Autodesk Inventor part; units mm, degrees
(part 5 of 6)
  line L3382 (247.1746, 190.2602) -> (246.7243, 190.3176)
  line L3383 (246.7243, 190.3176) -> (246.2809, 190.3966)
  line L3384 (246.2809, 190.3966) -> (245.8455, 190.4972)
  line L3385 (245.8455, 190.4972) -> (245.4186, 190.6185)
  line L3386 (245.4186, 190.6185) -> (245.0004, 190.7599)
  line L3387 (245.0004, 190.7599) -> (244.5914, 190.9212)
  line L3388 (244.5914, 190.9212) -> (244.1928, 191.1013)
  line L3389 (244.1928, 191.1013) -> (243.8049, 191.3001)
  line L3390 (243.8049, 191.3001) -> (243.428, 191.5168)
  line L3391 (243.428, 191.5168) -> (243.0629, 191.7509)
  line L3392 (243.0629, 191.7509) -> (242.7101, 192.0019)
  line L3393 (242.7101, 192.0019) -> (242.37, 192.2691)
  line L3394 (242.37, 192.2691) -> (242.0435, 192.5519)
  line L3395 (242.0435, 192.5519) -> (241.7306, 192.8499)
  line L3396 (241.7306, 192.8499) -> (241.433, 193.1624)
  line L3397 (241.433, 193.1624) -> (241.1498, 193.489)
  line L3398 (241.1498, 193.489) -> (240.8828, 193.829)
  line L3399 (240.8828, 193.829) -> (240.632, 194.1818)
  line L3400 (240.632, 194.1818) -> (240.3977, 194.547)
  line L3401 (240.3977, 194.547) -> (240.181, 194.9238)
  line L3402 (240.181, 194.9238) -> (239.9823, 195.3119)
  line L3403 (239.9823, 195.3119) -> (239.8021, 195.7107)
  line L3404 (239.8021, 195.7107) -> (239.6408, 196.1193)
  line L3405 (239.6408, 196.1193) -> (239.4992, 196.5375)
  line L3406 (239.4992, 196.5375) -> (239.378, 196.9645)
  line L3407 (239.378, 196.9645) -> (239.2777, 197.4)
  line L3408 (239.2777, 197.4) -> (239.1985, 197.8432)
  line L3409 (239.1985, 197.8432) -> (239.1413, 198.2937)
  line L3410 (239.1413, 198.2937) -> (239.1065, 198.7507)
  line L3411 (239.1065, 198.7507) -> (239.0948, 199.2139)
  line L3412 (239.0948, 171.1778) -> (239.1065, 171.641)
  line L3413 (239.1065, 171.641) -> (239.1413, 172.098)
  line L3414 (239.1413, 172.098) -> (239.1985, 172.5485)
  line L3415 (239.1985, 172.5485) -> (239.2777, 172.9917)
  line L3416 (239.2777, 172.9917) -> (239.378, 173.4271)
  line L3417 (239.378, 173.4271) -> (239.4992, 173.8542)
  line L3418 (239.4992, 173.8542) -> (239.6408, 174.2724)
  line L3419 (239.6408, 174.2724) -> (239.8021, 174.681)
  line L3420 (239.8021, 174.681) -> (239.9823, 175.0798)
  line L3421 (239.9823, 175.0798) -> (240.181, 175.4678)
  line L3422 (240.181, 175.4678) -> (240.3977, 175.8447)
  line L3423 (240.3977, 175.8447) -> (240.632, 176.2097)
  line L3424 (240.632, 176.2097) -> (240.8828, 176.5627)
  line L3425 (240.8828, 176.5627) -> (241.1498, 176.9027)
  line L3426 (241.1498, 176.9027) -> (241.433, 177.2291)
  line L3427 (241.433, 177.2291) -> (241.7306, 177.5418)
  line L3428 (241.7306, 177.5418) -> (242.0435, 177.8398)
  line L3429 (242.0435, 177.8398) -> (242.37, 178.1226)
  line L3430 (242.37, 178.1226) -> (242.7101, 178.3898)
  line L3431 (242.7101, 178.3898) -> (243.0629, 178.6408)
  line L3432 (243.0629, 178.6408) -> (243.428, 178.8749)
  line L3433 (243.428, 178.8749) -> (243.8049, 179.0916)
  line L3434 (243.8049, 179.0916) -> (244.1928, 179.2903)
  line L3435 (244.1928, 179.2903) -> (244.5914, 179.4705)
  line L3436 (244.5914, 179.4705) -> (245.0004, 179.6318)
  line L3437 (245.0004, 179.6318) -> (245.4186, 179.7732)
  line L3438 (245.4186, 179.7732) -> (245.8455, 179.8944)
  line L3439 (245.8455, 179.8944) -> (246.2809, 179.995)
  line L3440 (246.2809, 179.995) -> (246.7243, 180.0741)
  line L3441 (246.7243, 180.0741) -> (247.1746, 180.1313)
  line L3442 (247.1746, 180.1313) -> (247.6317, 180.1661)
  line L3443 (247.6317, 180.1661) -> (248.0948, 180.1778)
  line L3444 (248.0948, 180.1778) -> (248.5578, 180.1661)
  line L3445 (248.5578, 180.1661) -> (249.0149, 180.1313)
  line L3446 (249.0149, 180.1313) -> (249.4656, 180.0741)
  line L3447 (249.4656, 180.0741) -> (249.9086, 179.995)
  line L3448 (249.9086, 179.995) -> (250.3441, 179.8944)
  line L3449 (250.3441, 179.8944) -> (250.7713, 179.7732)
  line L3450 (250.7713, 179.7732) -> (251.1891, 179.6318)
  line L3451 (251.1891, 179.6318) -> (251.5981, 179.4705)
  line L3452 (251.5981, 179.4705) -> (251.9967, 179.2903)
  line L3453 (251.9967, 179.2903) -> (252.3846, 179.0916)
  line L3454 (252.3846, 179.0916) -> (252.7615, 178.8749)
  line L3455 (252.7615, 178.8749) -> (253.1267, 178.6408)
  line L3456 (253.1267, 178.6408) -> (253.4798, 178.3898)
  line L3457 (253.4798, 178.3898) -> (253.8195, 178.1226)
  line L3458 (253.8195, 178.1226) -> (254.1461, 177.8398)
  line L3459 (254.1461, 177.8398) -> (254.4589, 177.5418)
  line L3460 (254.4589, 177.5418) -> (254.7569, 177.2291)
  line L3461 (254.7569, 177.2291) -> (255.0397, 176.9027)
  line L3462 (255.0397, 176.9027) -> (255.3067, 176.5627)
  line L3463 (255.3067, 176.5627) -> (255.5579, 176.2097)
  line L3464 (255.5579, 176.2097) -> (255.7918, 175.8447)
  line L3465 (255.7918, 175.8447) -> (256.0085, 175.4678)
  line L3466 (256.0085, 175.4678) -> (256.2073, 175.0798)
  line L3467 (256.2073, 175.0798) -> (256.3875, 174.681)
  line L3468 (256.3875, 174.681) -> (256.5487, 174.2724)
  line L3469 (256.5487, 174.2724) -> (256.6903, 173.8542)
  line L3470 (256.6903, 173.8542) -> (256.8115, 173.4271)
  line L3471 (256.8115, 173.4271) -> (256.9118, 172.9917)
  line L3472 (256.9118, 172.9917) -> (256.991, 172.5485)
  line L3473 (256.991, 172.5485) -> (257.0482, 172.098)
  line L3474 (257.0482, 172.098) -> (257.083, 171.641)
  line L3475 (257.083, 171.641) -> (257.0947, 171.1778)
  line L3476 (257.0947, 171.1778) -> (257.083, 170.7146)
  line L3477 (257.083, 170.7146) -> (257.0482, 170.2577)
  line L3478 (257.0482, 170.2577) -> (256.991, 169.8072)
  line L3479 (256.991, 169.8072) -> (256.9118, 169.364)
  line L3480 (256.9118, 169.364) -> (256.8115, 168.9285)
  line L3481 (256.8115, 168.9285) -> (256.6903, 168.5015)
  line L3482 (256.6903, 168.5015) -> (256.5487, 168.0833)
  line L3483 (256.5487, 168.0833) -> (256.3875, 167.6747)
  line L3484 (256.3875, 167.6747) -> (256.2073, 167.2759)
  line L3485 (256.2073, 167.2759) -> (256.0085, 166.8878)
  line L3486 (256.0085, 166.8878) -> (255.7918, 166.5109)
  line L3487 (255.7918, 166.5109) -> (255.5579, 166.1459)
  line L3488 (255.5579, 166.1459) -> (255.3067, 165.793)
  line L3489 (255.3067, 165.793) -> (255.0397, 165.4529)
  line L3490 (255.0397, 165.4529) -> (254.7569, 165.1265)
  line L3491 (254.7569, 165.1265) -> (254.4589, 164.8139)
  line L3492 (254.4589, 164.8139) -> (254.1461, 164.5159)
  line L3493 (254.1461, 164.5159) -> (253.8195, 164.233)
  line L3494 (253.8195, 164.233) -> (253.4798, 163.9659)
  line L3495 (253.4798, 163.9659) -> (253.1267, 163.7149)
  line L3496 (253.1267, 163.7149) -> (252.7615, 163.4808)
  line L3497 (252.7615, 163.4808) -> (252.3846, 163.2641)
  line L3498 (252.3846, 163.2641) -> (251.9967, 163.0653)
  line L3499 (251.9967, 163.0653) -> (251.5981, 162.8851)
  line L3500 (251.5981, 162.8851) -> (251.1891, 162.7239)
  line L3501 (251.1891, 162.7239) -> (250.7713, 162.5825)
  line L3502 (250.7713, 162.5825) -> (250.3441, 162.4612)
  line L3503 (250.3441, 162.4612) -> (249.9086, 162.3606)
  line L3504 (249.9086, 162.3606) -> (249.4656, 162.2816)
  line L3505 (249.4656, 162.2816) -> (249.0149, 162.2244)
  line L3506 (249.0149, 162.2244) -> (248.5578, 162.1896)
  line L3507 (248.5578, 162.1896) -> (248.0948, 162.1779)
  line L3508 (248.0948, 162.1779) -> (247.6317, 162.1896)
  line L3509 (247.6317, 162.1896) -> (247.1746, 162.2244)
  line L3510 (247.1746, 162.2244) -> (246.7243, 162.2816)
  line L3511 (246.7243, 162.2816) -> (246.2809, 162.3606)
  line L3512 (246.2809, 162.3606) -> (245.8455, 162.4612)
  line L3513 (245.8455, 162.4612) -> (245.4186, 162.5825)
  line L3514 (245.4186, 162.5825) -> (245.0004, 162.7239)
  line L3515 (245.0004, 162.7239) -> (244.5914, 162.8851)
  line L3516 (244.5914, 162.8851) -> (244.1928, 163.0653)
  line L3517 (244.1928, 163.0653) -> (243.8049, 163.2641)
  line L3518 (243.8049, 163.2641) -> (243.428, 163.4808)
  line L3519 (243.428, 163.4808) -> (243.0629, 163.7149)
  line L3520 (243.0629, 163.7149) -> (242.7101, 163.9659)
  line L3521 (242.7101, 163.9659) -> (242.37, 164.233)
  line L3522 (242.37, 164.233) -> (242.0435, 164.5159)
  line L3523 (242.0435, 164.5159) -> (241.7306, 164.8139)
  line L3524 (241.7306, 164.8139) -> (241.433, 165.1265)
  line L3525 (241.433, 165.1265) -> (241.1498, 165.4529)
  line L3526 (241.1498, 165.4529) -> (240.8828, 165.793)
  line L3527 (240.8828, 165.793) -> (240.632, 166.1459)
  line L3528 (240.632, 166.1459) -> (240.3977, 166.5109)
  line L3529 (240.3977, 166.5109) -> (240.181, 166.8878)
  line L3530 (240.181, 166.8878) -> (239.9823, 167.2759)
  line L3531 (239.9823, 167.2759) -> (239.8021, 167.6747)
  line L3532 (239.8021, 167.6747) -> (239.6408, 168.0833)
  line L3533 (239.6408, 168.0833) -> (239.4992, 168.5015)
  line L3534 (239.4992, 168.5015) -> (239.378, 168.9285)
  line L3535 (239.378, 168.9285) -> (239.2777, 169.364)
  line L3536 (239.2777, 169.364) -> (239.1985, 169.8072)
  line L3537 (239.1985, 169.8072) -> (239.1413, 170.2577)
  line L3538 (239.1413, 170.2577) -> (239.1065, 170.7146)
  line L3539 (239.1065, 170.7146) -> (239.0948, 171.1778)
  line L3540 (242.0924, 148.6958) -> (242.1003, 149.0045)
  line L3541 (242.1003, 149.0045) -> (242.1234, 149.3092)
  line L3542 (242.1234, 149.3092) -> (242.1616, 149.6096)
  line L3543 (242.1616, 149.6096) -> (242.2143, 149.9051)
  line L3544 (242.2143, 149.9051) -> (242.3621, 150.48)
  line L3545 (242.3621, 150.48) -> (242.564, 151.0313)
  line L3546 (242.564, 151.0313) -> (242.8165, 151.5558)
  line L3547 (242.8165, 151.5558) -> (243.1169, 152.0505)
  line L3548 (243.1169, 152.0505) -> (243.4625, 152.5123)
  line L3549 (243.4625, 152.5123) -> (243.8497, 152.9385)
  line L3550 (243.8497, 152.9385) -> (244.2759, 153.3257)
  line L3551 (244.2759, 153.3257) -> (244.7379, 153.6711)
  line L3552 (244.7379, 153.6711) -> (245.2326, 153.9717)
  line L3553 (245.2326, 153.9717) -> (245.7569, 154.2244)
  line L3554 (245.7569, 154.2244) -> (246.3081, 154.4261)
  line L3555 (246.3081, 154.4261) -> (246.8831, 154.5739)
  line L3556 (246.8831, 154.5739) -> (247.1787, 154.6267)
  line L3557 (247.1787, 154.6267) -> (247.4788, 154.6648)
  line L3558 (247.4788, 154.6648) -> (247.7837, 154.6881)
  line L3559 (247.7837, 154.6881) -> (248.0924, 154.6958)
  line L3560 (248.0924, 154.6958) -> (248.401, 154.6881)
  line L3561 (248.401, 154.6881) -> (248.7059, 154.6648)
  line L3562 (248.7059, 154.6648) -> (249.006, 154.6267)
  line L3563 (249.006, 154.6267) -> (249.3016, 154.5739)
  line L3564 (249.3016, 154.5739) -> (249.8766, 154.4261)
  line L3565 (249.8766, 154.4261) -> (250.4278, 154.2244)
  line L3566 (250.4278, 154.2244) -> (250.9525, 153.9717)
  line L3567 (250.9525, 153.9717) -> (251.4472, 153.6711)
  line L3568 (251.4472, 153.6711) -> (251.9088, 153.3257)
  line L3569 (251.9088, 153.3257) -> (252.335, 152.9385)
  line L3570 (252.335, 152.9385) -> (252.7222, 152.5123)
  line L3571 (252.7222, 152.5123) -> (253.0678, 152.0505)
  line L3572 (253.0678, 152.0505) -> (253.3682, 151.5558)
  line L3573 (253.3682, 151.5558) -> (253.621, 151.0313)
  line L3574 (253.621, 151.0313) -> (253.8226, 150.48)
  line L3575 (253.8226, 150.48) -> (253.9704, 149.9051)
  line L3576 (253.9704, 149.9051) -> (254.0234, 149.6096)
  line L3577 (254.0234, 149.6096) -> (254.0613, 149.3092)
  line L3578 (254.0613, 149.3092) -> (254.0847, 149.0045)
  line L3579 (254.0847, 149.0045) -> (254.0923, 148.6958)
  line L3580 (254.0923, 148.6958) -> (254.0847, 148.3872)
  line L3581 (254.0847, 148.3872) -> (254.0613, 148.0823)
  line L3582 (254.0613, 148.0823) -> (254.0234, 147.7822)
  line L3583 (254.0234, 147.7822) -> (253.9704, 147.4866)
  line L3584 (253.9704, 147.4866) -> (253.8226, 146.9116)
  line L3585 (253.8226, 146.9116) -> (253.621, 146.3604)
  line L3586 (253.621, 146.3604) -> (253.3682, 145.8357)
  line L3587 (253.3682, 145.8357) -> (253.0678, 145.341)
  line L3588 (253.0678, 145.341) -> (252.7222, 144.8794)
  line L3589 (252.7222, 144.8794) -> (252.335, 144.4532)
  line L3590 (252.335, 144.4532) -> (251.9088, 144.066)
  line L3591 (251.9088, 144.066) -> (251.4472, 143.7204)
  line L3592 (251.4472, 143.7204) -> (250.9525, 143.42)
  line L3593 (250.9525, 143.42) -> (250.4278, 143.1675)
  line L3594 (250.4278, 143.1675) -> (249.8766, 142.9656)
  line L3595 (249.8766, 142.9656) -> (249.3016, 142.8178)
  line L3596 (249.3016, 142.8178) -> (249.006, 142.7651)
  line L3597 (249.006, 142.7651) -> (248.7059, 142.7269)
  line L3598 (248.7059, 142.7269) -> (248.401, 142.7038)
  line L3599 (248.401, 142.7038) -> (248.0924, 142.6959)
  line L3600 (248.0924, 142.6959) -> (247.7837, 142.7038)
  line L3601 (247.7837, 142.7038) -> (247.4788, 142.7269)
  line L3602 (247.4788, 142.7269) -> (247.1787, 142.7651)
  line L3603 (247.1787, 142.7651) -> (246.8831, 142.8178)
  line L3604 (246.8831, 142.8178) -> (246.3081, 142.9656)
  line L3605 (246.3081, 142.9656) -> (245.7569, 143.1675)
  line L3606 (245.7569, 143.1675) -> (245.2326, 143.42)
  line L3607 (245.2326, 143.42) -> (244.7379, 143.7204)
  line L3608 (244.7379, 143.7204) -> (244.2759, 144.066)
  line L3609 (244.2759, 144.066) -> (243.8497, 144.4532)
  line L3610 (243.8497, 144.4532) -> (243.4625, 144.8794)
  line L3611 (243.4625, 144.8794) -> (243.1169, 145.341)
  line L3612 (243.1169, 145.341) -> (242.8165, 145.8357)
  line L3613 (242.8165, 145.8357) -> (242.564, 146.3604)
  line L3614 (242.564, 146.3604) -> (242.3621, 146.9116)
  line L3615 (242.3621, 146.9116) -> (242.2143, 147.4866)
  line L3616 (242.2143, 147.4866) -> (242.1616, 147.7822)
  line L3617 (242.1616, 147.7822) -> (242.1234, 148.0823)
  line L3618 (242.1234, 148.0823) -> (242.1003, 148.3872)
  line L3619 (242.1003, 148.3872) -> (242.0924, 148.6958)
  line L3620 (239.0948, 126.1997) -> (239.1065, 126.6631)
  line L3621 (239.1065, 126.6631) -> (239.1413, 127.1199)
  line L3622 (239.1413, 127.1199) -> (239.1985, 127.5705)
  line L3623 (239.1985, 127.5705) -> (239.2777, 128.0135)
  line L3624 (239.2777, 128.0135) -> (239.378, 128.449)
  line L3625 (239.378, 128.449) -> (239.4992, 128.8762)
  line L3626 (239.4992, 128.8762) -> (239.6408, 129.2944)
  line L3627 (239.6408, 129.2944) -> (239.8021, 129.703)
  line L3628 (239.8021, 129.703) -> (239.9823, 130.1016)
  line L3629 (239.9823, 130.1016) -> (240.181, 130.4899)
  line L3630 (240.181, 130.4899) -> (240.3977, 130.8668)
  line L3631 (240.3977, 130.8668) -> (240.632, 131.232)
  line L3632 (240.632, 131.232) -> (240.8828, 131.5847)
  line L3633 (240.8828, 131.5847) -> (241.1498, 131.9248)
  line L3634 (241.1498, 131.9248) -> (241.433, 132.2514)
  line L3635 (241.433, 132.2514) -> (241.7306, 132.5638)
  line L3636 (241.7306, 132.5638) -> (242.0435, 132.8618)
  line L3637 (242.0435, 132.8618) -> (242.37, 133.1447)
  line L3638 (242.37, 133.1447) -> (242.7101, 133.412)
  line L3639 (242.7101, 133.412) -> (243.0629, 133.6628)
  line L3640 (243.0629, 133.6628) -> (243.428, 133.8967)
  line L3641 (243.428, 133.8967) -> (243.8049, 134.1134)
  line L3642 (243.8049, 134.1134) -> (244.1928, 134.3122)
  line L3643 (244.1928, 134.3122) -> (244.5914, 134.4924)
  line L3644 (244.5914, 134.4924) -> (245.0004, 134.6536)
  line L3645 (245.0004, 134.6536) -> (245.4186, 134.7952)
  line L3646 (245.4186, 134.7952) -> (245.8455, 134.9165)
  line L3647 (245.8455, 134.9165) -> (246.2809, 135.0171)
  line L3648 (246.2809, 135.0171) -> (246.7243, 135.096)
  line L3649 (246.7243, 135.096) -> (247.1746, 135.1535)
  line L3650 (247.1746, 135.1535) -> (247.6317, 135.188)
  line L3651 (247.6317, 135.188) -> (248.0948, 135.1997)
  line L3652 (248.0948, 135.1997) -> (248.5578, 135.188)
  line L3653 (248.5578, 135.188) -> (249.0149, 135.1535)
  line L3654 (249.0149, 135.1535) -> (249.4656, 135.096)
  line L3655 (249.4656, 135.096) -> (249.9086, 135.0171)
  line L3656 (249.9086, 135.0171) -> (250.3441, 134.9165)
  line L3657 (250.3441, 134.9165) -> (250.7713, 134.7952)
  line L3658 (250.7713, 134.7952) -> (251.1891, 134.6536)
  line L3659 (251.1891, 134.6536) -> (251.5981, 134.4924)
  line L3660 (251.5981, 134.4924) -> (251.9967, 134.3122)
  line L3661 (251.9967, 134.3122) -> (252.3846, 134.1134)
  line L3662 (252.3846, 134.1134) -> (252.7615, 133.8967)
  line L3663 (252.7615, 133.8967) -> (253.1267, 133.6628)
  line L3664 (253.1267, 133.6628) -> (253.4798, 133.412)
  line L3665 (253.4798, 133.412) -> (253.8195, 133.1447)
  line L3666 (253.8195, 133.1447) -> (254.1461, 132.8618)
  line L3667 (254.1461, 132.8618) -> (254.4589, 132.5638)
  line L3668 (254.4589, 132.5638) -> (254.7569, 132.2514)
  line L3669 (254.7569, 132.2514) -> (255.0397, 131.9248)
  line L3670 (255.0397, 131.9248) -> (255.3067, 131.5847)
  line L3671 (255.3067, 131.5847) -> (255.5579, 131.232)
  line L3672 (255.5579, 131.232) -> (255.7918, 130.8668)
  line L3673 (255.7918, 130.8668) -> (256.0085, 130.4899)
  line L3674 (256.0085, 130.4899) -> (256.2073, 130.1016)
  line L3675 (256.2073, 130.1016) -> (256.3875, 129.703)
  line L3676 (256.3875, 129.703) -> (256.5487, 129.2944)
  line L3677 (256.5487, 129.2944) -> (256.6903, 128.8762)
  line L3678 (256.6903, 128.8762) -> (256.8115, 128.449)
  line L3679 (256.8115, 128.449) -> (256.9118, 128.0135)
  line L3680 (256.9118, 128.0135) -> (256.991, 127.5705)
  line L3681 (256.991, 127.5705) -> (257.0482, 127.1199)
  line L3682 (257.0482, 127.1199) -> (257.083, 126.6631)
  line L3683 (257.083, 126.6631) -> (257.0947, 126.1997)
  line L3684 (257.0947, 126.1997) -> (257.083, 125.7367)
  line L3685 (257.083, 125.7367) -> (257.0482, 125.2795)
  line L3686 (257.0482, 125.2795) -> (256.991, 124.8292)
  line L3687 (256.991, 124.8292) -> (256.9118, 124.3859)
  line L3688 (256.9118, 124.3859) -> (256.8115, 123.9507)
  line L3689 (256.8115, 123.9507) -> (256.6903, 123.5236)
  line L3690 (256.6903, 123.5236) -> (256.5487, 123.1053)
  line L3691 (256.5487, 123.1053) -> (256.3875, 122.6967)
  line L3692 (256.3875, 122.6967) -> (256.2073, 122.2981)
  line L3693 (256.2073, 122.2981) -> (256.0085, 121.9099)
  line L3694 (256.0085, 121.9099) -> (255.7918, 121.533)
  line L3695 (255.7918, 121.533) -> (255.5579, 121.1678)
  line L3696 (255.5579, 121.1678) -> (255.3067, 120.815)
  line L3697 (255.3067, 120.815) -> (255.0397, 120.475)
  line L3698 (255.0397, 120.475) -> (254.7569, 120.1484)
  line L3699 (254.7569, 120.1484) -> (254.4589, 119.8359)
  line L3700 (254.4589, 119.8359) -> (254.1461, 119.5379)
  line L3701 (254.1461, 119.5379) -> (253.8195, 119.2551)
  line L3702 (253.8195, 119.2551) -> (253.4798, 118.9877)
  line L3703 (253.4798, 118.9877) -> (253.1267, 118.7369)
  line L3704 (253.1267, 118.7369) -> (252.7615, 118.5027)
  line L3705 (252.7615, 118.5027) -> (252.3846, 118.286)
  line L3706 (252.3846, 118.286) -> (251.9967, 118.0872)
  line L3707 (251.9967, 118.0872) -> (251.5981, 117.907)
  line L3708 (251.5981, 117.907) -> (251.1891, 117.7458)
  line L3709 (251.1891, 117.7458) -> (250.7713, 117.6045)
  line L3710 (250.7713, 117.6045) -> (250.3441, 117.4833)
  line L3711 (250.3441, 117.4833) -> (249.9086, 117.3827)
  line L3712 (249.9086, 117.3827) -> (249.4656, 117.3034)
  line L3713 (249.4656, 117.3034) -> (249.0149, 117.2462)
  line L3714 (249.0149, 117.2462) -> (248.5578, 117.2115)
  line L3715 (248.5578, 117.2115) -> (248.0948, 117.1997)
  line L3716 (248.0948, 117.1997) -> (247.6317, 117.2115)
  line L3717 (247.6317, 117.2115) -> (247.1746, 117.2462)
  line L3718 (247.1746, 117.2462) -> (246.7243, 117.3034)
  line L3719 (246.7243, 117.3034) -> (246.2809, 117.3827)
  line L3720 (246.2809, 117.3827) -> (245.8455, 117.4833)
  line L3721 (245.8455, 117.4833) -> (245.4186, 117.6045)
  line L3722 (245.4186, 117.6045) -> (245.0004, 117.7458)
  line L3723 (245.0004, 117.7458) -> (244.5914, 117.907)
  line L3724 (244.5914, 117.907) -> (244.1928, 118.0872)
  line L3725 (244.1928, 118.0872) -> (243.8049, 118.286)
  line L3726 (243.8049, 118.286) -> (243.428, 118.5027)
  line L3727 (243.428, 118.5027) -> (243.0629, 118.7369)
  line L3728 (243.0629, 118.7369) -> (242.7101, 118.9877)
  line L3729 (242.7101, 118.9877) -> (242.37, 119.2551)
  line L3730 (242.37, 119.2551) -> (242.0435, 119.5379)
  line L3731 (242.0435, 119.5379) -> (241.7306, 119.8359)
  line L3732 (241.7306, 119.8359) -> (241.433, 120.1484)
  line L3733 (241.433, 120.1484) -> (241.1498, 120.475)
  line L3734 (241.1498, 120.475) -> (240.8828, 120.815)
  line L3735 (240.8828, 120.815) -> (240.632, 121.1678)
  line L3736 (240.632, 121.1678) -> (240.3977, 121.533)
  line L3737 (240.3977, 121.533) -> (240.181, 121.9099)
  line L3738 (240.181, 121.9099) -> (239.9823, 122.2981)
  line L3739 (239.9823, 122.2981) -> (239.8021, 122.6967)
  line L3740 (239.8021, 122.6967) -> (239.6408, 123.1053)
  line L3741 (239.6408, 123.1053) -> (239.4992, 123.5236)
  line L3742 (239.4992, 123.5236) -> (239.378, 123.9507)
  line L3743 (239.378, 123.9507) -> (239.2777, 124.3859)
  line L3744 (239.2777, 124.3859) -> (239.1985, 124.8292)
  line L3745 (239.1985, 124.8292) -> (239.1413, 125.2795)
  line L3746 (239.1413, 125.2795) -> (239.1065, 125.7367)
  line L3747 (239.1065, 125.7367) -> (239.0948, 126.1997)
  line L3748 (239.0755, 98.1797) -> (239.0872, 98.6431)
  line L3749 (239.0872, 98.6431) -> (239.122, 99.0999)
  line L3750 (239.122, 99.0999) -> (239.1792, 99.5505)
  line L3751 (239.1792, 99.5505) -> (239.2584, 99.9936)
  line L3752 (239.2584, 99.9936) -> (239.3587, 100.429)
  line L3753 (239.3587, 100.429) -> (239.48, 100.8562)
  line L3754 (239.48, 100.8562) -> (239.6215, 101.2744)
  line L3755 (239.6215, 101.2744) -> (239.7828, 101.683)
  line L3756 (239.7828, 101.683) -> (239.963, 102.0816)
  line L3757 (239.963, 102.0816) -> (240.1617, 102.4699)
  line L3758 (240.1617, 102.4699) -> (240.3784, 102.8468)
  line L3759 (240.3784, 102.8468) -> (240.6124, 103.212)
  line L3760 (240.6124, 103.212) -> (240.8635, 103.5647)
  line L3761 (240.8635, 103.5647) -> (241.1305, 103.9048)
  line L3762 (241.1305, 103.9048) -> (241.4133, 104.2314)
  line L3763 (241.4133, 104.2314) -> (241.7113, 104.5438)
  line L3764 (241.7113, 104.5438) -> (242.0242, 104.8418)
  line L3765 (242.0242, 104.8418) -> (242.3508, 105.1247)
  line L3766 (242.3508, 105.1247) -> (242.6904, 105.392)
  line L3767 (242.6904, 105.392) -> (243.0436, 105.6428)
  line L3768 (243.0436, 105.6428) -> (243.4084, 105.8767)
  line L3769 (243.4084, 105.8767) -> (243.7853, 106.0934)
  line L3770 (243.7853, 106.0934) -> (244.1736, 106.2922)
  line L3771 (244.1736, 106.2922) -> (244.5722, 106.4727)
  line L3772 (244.5722, 106.4727) -> (244.9807, 106.6336)
  line L3773 (244.9807, 106.6336) -> (245.399, 106.7752)
  line L3774 (245.399, 106.7752) -> (245.8262, 106.8965)
  line L3775 (245.8262, 106.8965) -> (246.2616, 106.9971)
  line L3776 (246.2616, 106.9971) -> (246.7047, 107.076)
  line L3777 (246.7047, 107.076) -> (247.1553, 107.1335)
  line L3778 (247.1553, 107.1335) -> (247.6121, 107.168)
  line L3779 (247.6121, 107.168) -> (248.0755, 107.1797)
  line L3780 (248.0755, 107.1797) -> (248.5385, 107.168)
  line L3781 (248.5385, 107.168) -> (248.9957, 107.1335)
  line L3782 (248.9957, 107.1335) -> (249.4459, 107.076)
  line L3783 (249.4459, 107.076) -> (249.8893, 106.9971)
  line L3784 (249.8893, 106.9971) -> (250.3248, 106.8965)
  line L3785 (250.3248, 106.8965) -> (250.7516, 106.7752)
  line L3786 (250.7516, 106.7752) -> (251.1699, 106.6336)
  line L3787 (251.1699, 106.6336) -> (251.5788, 106.4727)
  line L3788 (251.5788, 106.4727) -> (251.9774, 106.2922)
  line L3789 (251.9774, 106.2922) -> (252.3653, 106.0934)
  line L3790 (252.3653, 106.0934) -> (252.7422, 105.8767)
  line L3791 (252.7422, 105.8767) -> (253.1074, 105.6428)
  line L3792 (253.1074, 105.6428) -> (253.4602, 105.392)
  line L3793 (253.4602, 105.392) -> (253.8002, 105.1247)
  line L3794 (253.8002, 105.1247) -> (254.1268, 104.8418)
  line L3795 (254.1268, 104.8418) -> (254.4392, 104.5438)
  line L3796 (254.4392, 104.5438) -> (254.7373, 104.2314)
  line L3797 (254.7373, 104.2314) -> (255.0201, 103.9048)
  line L3798 (255.0201, 103.9048) -> (255.2874, 103.5647)
  line L3799 (255.2874, 103.5647) -> (255.5382, 103.212)
  line L3800 (255.5382, 103.212) -> (255.7725, 102.8468)
  line L3801 (255.7725, 102.8468) -> (255.9892, 102.4699)
  line L3802 (255.9892, 102.4699) -> (256.188, 102.0816)
  line L3803 (256.188, 102.0816) -> (256.3682, 101.683)
  line L3804 (256.3682, 101.683) -> (256.5294, 101.2744)
  line L3805 (256.5294, 101.2744) -> (256.6706, 100.8562)
  line L3806 (256.6706, 100.8562) -> (256.7919, 100.429)
  line L3807 (256.7919, 100.429) -> (256.8925, 99.9936)
  line L3808 (256.8925, 99.9936) -> (256.9717, 99.5505)
  line L3809 (256.9717, 99.5505) -> (257.0289, 99.0999)
  line L3810 (257.0289, 99.0999) -> (257.0637, 98.6431)
  line L3811 (257.0637, 98.6431) -> (257.0754, 98.1797)
  line L3812 (257.0754, 98.1797) -> (257.0637, 97.7167)
  line L3813 (257.0637, 97.7167) -> (257.0289, 97.2595)
  line L3814 (257.0289, 97.2595) -> (256.9717, 96.8093)
  line L3815 (256.9717, 96.8093) -> (256.8925, 96.3659)
  line L3816 (256.8925, 96.3659) -> (256.7919, 95.9308)
  line L3817 (256.7919, 95.9308) -> (256.6706, 95.5036)
  line L3818 (256.6706, 95.5036) -> (256.5294, 95.0853)
  line L3819 (256.5294, 95.0853) -> (256.3682, 94.6767)
  line L3820 (256.3682, 94.6767) -> (256.188, 94.2778)
  line L3821 (256.188, 94.2778) -> (255.9892, 93.8899)
  line L3822 (255.9892, 93.8899) -> (255.7725, 93.513)
  line L3823 (255.7725, 93.513) -> (255.5382, 93.1478)
  line L3824 (255.5382, 93.1478) -> (255.2874, 92.795)
  line L3825 (255.2874, 92.795) -> (255.0201, 92.455)
  line L3826 (255.0201, 92.455) -> (254.7373, 92.1284)
  line L3827 (254.7373, 92.1284) -> (254.4392, 91.8159)
  line L3828 (254.4392, 91.8159) -> (254.1268, 91.5179)
  line L3829 (254.1268, 91.5179) -> (253.8002, 91.2351)
  line L3830 (253.8002, 91.2351) -> (253.4602, 90.9677)
  line L3831 (253.4602, 90.9677) -> (253.1074, 90.7169)
  line L3832 (253.1074, 90.7169) -> (252.7422, 90.4827)
  line L3833 (252.7422, 90.4827) -> (252.3653, 90.266)
  line L3834 (252.3653, 90.266) -> (251.9774, 90.0672)
  line L3835 (251.9774, 90.0672) -> (251.5788, 89.887)
  line L3836 (251.5788, 89.887) -> (251.1699, 89.7258)
  line L3837 (251.1699, 89.7258) -> (250.7516, 89.5845)
  line L3838 (250.7516, 89.5845) -> (250.3248, 89.4633)
  line L3839 (250.3248, 89.4633) -> (249.8893, 89.3627)
  line L3840 (249.8893, 89.3627) -> (249.4459, 89.2834)
  line L3841 (249.4459, 89.2834) -> (248.9957, 89.2263)
  line L3842 (248.9957, 89.2263) -> (248.5385, 89.1915)
  line L3843 (248.5385, 89.1915) -> (248.0755, 89.1797)
  line L3844 (248.0755, 89.1797) -> (247.6121, 89.1915)
  line L3845 (247.6121, 89.1915) -> (247.1553, 89.2263)
  line L3846 (247.1553, 89.2263) -> (246.7047, 89.2834)
  line L3847 (246.7047, 89.2834) -> (246.2616, 89.3627)
  line L3848 (246.2616, 89.3627) -> (245.8262, 89.4633)
  line L3849 (245.8262, 89.4633) -> (245.399, 89.5845)
  line L3850 (245.399, 89.5845) -> (244.9807, 89.7258)
  line L3851 (244.9807, 89.7258) -> (244.5722, 89.887)
  line L3852 (244.5722, 89.887) -> (244.1736, 90.0672)
  line L3853 (244.1736, 90.0672) -> (243.7853, 90.266)
  line L3854 (243.7853, 90.266) -> (243.4084, 90.4827)
  line L3855 (243.4084, 90.4827) -> (243.0436, 90.7169)
  line L3856 (243.0436, 90.7169) -> (242.6904, 90.9677)
  line L3857 (242.6904, 90.9677) -> (242.3508, 91.2351)
  line L3858 (242.3508, 91.2351) -> (242.0242, 91.5179)
  line L3859 (242.0242, 91.5179) -> (241.7113, 91.8159)
  line L3860 (241.7113, 91.8159) -> (241.4133, 92.1284)
  line L3861 (241.4133, 92.1284) -> (241.1305, 92.455)
  line L3862 (241.1305, 92.455) -> (240.8635, 92.795)
  line L3863 (240.8635, 92.795) -> (240.6124, 93.1478)
  line L3864 (240.6124, 93.1478) -> (240.3784, 93.513)
  line L3865 (240.3784, 93.513) -> (240.1617, 93.8899)
  line L3866 (240.1617, 93.8899) -> (239.963, 94.2778)
  line L3867 (239.963, 94.2778) -> (239.7828, 94.6767)
  line L3868 (239.7828, 94.6767) -> (239.6215, 95.0853)
  line L3869 (239.6215, 95.0853) -> (239.48, 95.5036)
  line L3870 (239.48, 95.5036) -> (239.3587, 95.9308)
  line L3871 (239.3587, 95.9308) -> (239.2584, 96.3659)
  line L3872 (239.2584, 96.3659) -> (239.1792, 96.8093)
  line L3873 (239.1792, 96.8093) -> (239.122, 97.2595)
  line L3874 (239.122, 97.2595) -> (239.0872, 97.7167)
  line L3875 (239.0872, 97.7167) -> (239.0755, 98.1797)
  line L3876 (264.5279, 87.8958) -> (264.5437, 88.2127)
  line L3877 (264.5437, 88.2127) -> (264.5909, 88.5207)
  line L3878 (264.5909, 88.5207) -> (264.667, 88.8177)
  line L3879 (264.667, 88.8177) -> (264.7714, 89.1026)
  line L3880 (264.7714, 89.1026) -> (264.902, 89.3734)
  line L3881 (264.902, 89.3734) -> (265.0574, 89.629)
  line L3882 (265.0574, 89.629) -> (265.2358, 89.8677)
  line L3883 (265.2358, 89.8677) -> (265.4356, 90.0879)
  line L3884 (265.4356, 90.0879) -> (265.6558, 90.288)
  line L3885 (265.6558, 90.288) -> (265.8945, 90.4665)
  line L3886 (265.8945, 90.4665) -> (266.1502, 90.6215)
  line L3887 (266.1502, 90.6215) -> (266.4209, 90.7521)
  line L3888 (266.4209, 90.7521) -> (266.7059, 90.8565)
  line L3889 (266.7059, 90.8565) -> (267.0032, 90.933)
  line L3890 (267.0032, 90.933) -> (267.3108, 90.9798)
  line L3891 (267.3108, 90.9798) -> (267.6278, 90.996)
  line L3892 (267.6278, 90.996) -> (267.9447, 90.9798)
  line L3893 (267.9447, 90.9798) -> (268.2524, 90.933)
  line L3894 (268.2524, 90.933) -> (268.5497, 90.8565)
  line L3895 (268.5497, 90.8565) -> (268.8346, 90.7521)
  line L3896 (268.8346, 90.7521) -> (269.1054, 90.6215)
  line L3897 (269.1054, 90.6215) -> (269.361, 90.4665)
  line L3898 (269.361, 90.4665) -> (269.5997, 90.288)
  line L3899 (269.5997, 90.288) -> (269.8199, 90.0879)
  line L3900 (269.8199, 90.0879) -> (270.02, 89.8677)
  line L3901 (270.02, 89.8677) -> (270.1985, 89.629)
  line L3902 (270.1985, 89.629) -> (270.3535, 89.3734)
  line L3903 (270.3535, 89.3734) -> (270.4841, 89.1026)
  line L3904 (270.4841, 89.1026) -> (270.5885, 88.8177)
  line L3905 (270.5885, 88.8177) -> (270.6646, 88.5207)
  line L3906 (270.6646, 88.5207) -> (270.7118, 88.2127)
  line L3907 (270.7118, 88.2127) -> (270.7277, 87.8958)
  line L3908 (270.7277, 87.8958) -> (270.7118, 87.5788)
  line L3909 (270.7118, 87.5788) -> (270.6646, 87.2712)
  line L3910 (270.6646, 87.2712) -> (270.5885, 86.9738)
  line L3911 (270.5885, 86.9738) -> (270.4841, 86.6893)
  line L3912 (270.4841, 86.6893) -> (270.3535, 86.4182)
  line L3913 (270.3535, 86.4182) -> (270.1985, 86.1625)
  line L3914 (270.1985, 86.1625) -> (270.02, 85.9238)
  line L3915 (270.02, 85.9238) -> (269.8199, 85.7036)
  line L3916 (269.8199, 85.7036) -> (269.5997, 85.5038)
  line L3917 (269.5997, 85.5038) -> (269.361, 85.3254)
  line L3918 (269.361, 85.3254) -> (269.1054, 85.17)
  line L3919 (269.1054, 85.17) -> (268.8346, 85.0394)
  line L3920 (268.8346, 85.0394) -> (268.5497, 84.935)
  line L3921 (268.5497, 84.935) -> (268.2524, 84.8589)
  line L3922 (268.2524, 84.8589) -> (267.9447, 84.8117)
  line L3923 (267.9447, 84.8117) -> (267.6278, 84.7959)
  line L3924 (267.6278, 84.7959) -> (267.3108, 84.8117)
  line L3925 (267.3108, 84.8117) -> (267.0032, 84.8589)
  line L3926 (267.0032, 84.8589) -> (266.7059, 84.935)
  line L3927 (266.7059, 84.935) -> (266.4209, 85.0394)
  line L3928 (266.4209, 85.0394) -> (266.1502, 85.17)
  line L3929 (266.1502, 85.17) -> (265.8945, 85.3254)
  line L3930 (265.8945, 85.3254) -> (265.6558, 85.5038)
  line L3931 (265.6558, 85.5038) -> (265.4356, 85.7036)
  line L3932 (265.4356, 85.7036) -> (265.2358, 85.9238)
  line L3933 (265.2358, 85.9238) -> (265.0574, 86.1625)
  line L3934 (265.0574, 86.1625) -> (264.902, 86.4182)
  line L3935 (264.902, 86.4182) -> (264.7714, 86.6893)
  line L3936 (264.7714, 86.6893) -> (264.667, 86.9738)
  line L3937 (264.667, 86.9738) -> (264.5909, 87.2712)
  line L3938 (264.5909, 87.2712) -> (264.5437, 87.5788)
  line L3939 (264.5437, 87.5788) -> (264.5279, 87.8958)
  line L3940 (264.5268, 148.6958) -> (264.5427, 149.0128)
  line L3941 (264.5427, 149.0128) -> (264.5899, 149.3206)
  line L3942 (264.5899, 149.3206) -> (264.666, 149.6177)
  line L3943 (264.666, 149.6177) -> (264.7704, 149.9025)
  line L3944 (264.7704, 149.9025) -> (264.901, 150.1734)
  line L3945 (264.901, 150.1734) -> (265.0563, 150.4291)
  line L3946 (265.0563, 150.4291) -> (265.2348, 150.6678)
  line L3947 (265.2348, 150.6678) -> (265.4346, 150.8879)
  line L3948 (265.4346, 150.8879) -> (265.6548, 151.0879)
  line L3949 (265.6548, 151.0879) -> (265.8935, 151.2664)
  line L3950 (265.8935, 151.2664) -> (266.1491, 151.4216)
  line L3951 (266.1491, 151.4216) -> (266.4203, 151.5522)
  line L3952 (266.4203, 151.5522) -> (266.7048, 151.6565)
  line L3953 (266.7048, 151.6565) -> (267.0021, 151.7329)
  line L3954 (267.0021, 151.7329) -> (267.3098, 151.7799)
  line L3955 (267.3098, 151.7799) -> (267.6267, 151.7959)
  line L3956 (267.6267, 151.7959) -> (267.9437, 151.7799)
  line L3957 (267.9437, 151.7799) -> (268.2517, 151.7329)
  line L3958 (268.2517, 151.7329) -> (268.5486, 151.6565)
  line L3959 (268.5486, 151.6565) -> (268.8335, 151.5522)
  line L3960 (268.8335, 151.5522) -> (269.1043, 151.4216)
  line L3961 (269.1043, 151.4216) -> (269.36, 151.2664)
  line L3962 (269.36, 151.2664) -> (269.5987, 151.0879)
  line L3963 (269.5987, 151.0879) -> (269.8188, 150.8879)
  line L3964 (269.8188, 150.8879) -> (270.019, 150.6678)
  line L3965 (270.019, 150.6678) -> (270.1975, 150.4291)
  line L3966 (270.1975, 150.4291) -> (270.3525, 150.1734)
  line L3967 (270.3525, 150.1734) -> (270.4831, 149.9025)
  line L3968 (270.4831, 149.9025) -> (270.5874, 149.6177)
  line L3969 (270.5874, 149.6177) -> (270.6639, 149.3206)
  line L3970 (270.6639, 149.3206) -> (270.7108, 149.0128)
  line L3971 (270.7108, 149.0128) -> (270.7266, 148.6958)
  line L3972 (270.7266, 148.6958) -> (270.7108, 148.3789)
  line L3973 (270.7108, 148.3789) -> (270.6639, 148.0712)
  line L3974 (270.6639, 148.0712) -> (270.5874, 147.7739)
  line L3975 (270.5874, 147.7739) -> (270.4831, 147.489)
  line L3976 (270.4831, 147.489) -> (270.3525, 147.2182)
  line L3977 (270.3525, 147.2182) -> (270.1975, 146.9626)
  line L3978 (270.1975, 146.9626) -> (270.019, 146.7239)
  line L3979 (270.019, 146.7239) -> (269.8188, 146.5037)
  line L3980 (269.8188, 146.5037) -> (269.5987, 146.3036)
  line L3981 (269.5987, 146.3036) -> (269.36, 146.1251)
  line L3982 (269.36, 146.1251) -> (269.1043, 145.9701)
  line L3983 (269.1043, 145.9701) -> (268.8335, 145.8395)
  line L3984 (268.8335, 145.8395) -> (268.5486, 145.7351)
  line L3985 (268.5486, 145.7351) -> (268.2517, 145.6586)
  line L3986 (268.2517, 145.6586) -> (267.9437, 145.6118)
  line L3987 (267.9437, 145.6118) -> (267.6267, 145.5959)
  line L3988 (267.6267, 145.5959) -> (267.3098, 145.6118)
  line L3989 (267.3098, 145.6118) -> (267.0021, 145.6586)
  line L3990 (267.0021, 145.6586) -> (266.7048, 145.7351)
  line L3991 (266.7048, 145.7351) -> (266.4203, 145.8395)
  line L3992 (266.4203, 145.8395) -> (266.1491, 145.9701)
  line L3993 (266.1491, 145.9701) -> (265.8935, 146.1251)
  line L3994 (265.8935, 146.1251) -> (265.6548, 146.3036)
  line L3995 (265.6548, 146.3036) -> (265.4346, 146.5037)
  line L3996 (265.4346, 146.5037) -> (265.2348, 146.7239)
  line L3997 (265.2348, 146.7239) -> (265.0563, 146.9626)
  line L3998 (265.0563, 146.9626) -> (264.901, 147.2182)
  line L3999 (264.901, 147.2182) -> (264.7704, 147.489)
  line L4000 (264.7704, 147.489) -> (264.666, 147.7739)
  line L4001 (264.666, 147.7739) -> (264.5899, 148.0712)
  line L4002 (264.5899, 148.0712) -> (264.5427, 148.3789)
  line L4003 (264.5427, 148.3789) -> (264.5268, 148.6958)
  line L4004 (264.5268, 209.4968) -> (264.5427, 209.8137)
  line L4005 (264.5427, 209.8137) -> (264.5899, 210.1215)
  line L4006 (264.5899, 210.1215) -> (264.666, 210.4187)
  line L4007 (264.666, 210.4187) -> (264.7704, 210.7034)
  line L4008 (264.7704, 210.7034) -> (264.901, 210.9745)
  line L4009 (264.901, 210.9745) -> (265.0563, 211.23)
  line L4010 (265.0563, 211.23) -> (265.2348, 211.4687)
  line L4011 (265.2348, 211.4687) -> (265.4346, 211.6889)
  line L4012 (265.4346, 211.6889) -> (265.6548, 211.8889)
  line L4013 (265.6548, 211.8889) -> (265.8935, 212.0673)
  line L4014 (265.8935, 212.0673) -> (266.1491, 212.2227)
  line L4015 (266.1491, 212.2227) -> (266.4203, 212.3533)
  line L4016 (266.4203, 212.3533) -> (266.7048, 212.4575)
  line L4017 (266.7048, 212.4575) -> (267.0021, 212.5338)
  line L4018 (267.0021, 212.5338) -> (267.3098, 212.5808)
  line L4019 (267.3098, 212.5808) -> (267.6267, 212.5968)
  line L4020 (267.6267, 212.5968) -> (267.9437, 212.5808)
  line L4021 (267.9437, 212.5808) -> (268.2517, 212.5338)
  line L4022 (268.2517, 212.5338) -> (268.5486, 212.4575)
  line L4023 (268.5486, 212.4575) -> (268.8335, 212.3533)
  line L4024 (268.8335, 212.3533) -> (269.1043, 212.2227)
  line L4025 (269.1043, 212.2227) -> (269.36, 212.0673)
  line L4026 (269.36, 212.0673) -> (269.5987, 211.8889)
  line L4027 (269.5987, 211.8889) -> (269.8188, 211.6889)
  line L4028 (269.8188, 211.6889) -> (270.019, 211.4687)
  line L4029 (270.019, 211.4687) -> (270.1975, 211.23)
  line L4030 (270.1975, 211.23) -> (270.3525, 210.9745)
  line L4031 (270.3525, 210.9745) -> (270.4831, 210.7034)
  line L4032 (270.4831, 210.7034) -> (270.5874, 210.4187)
  line L4033 (270.5874, 210.4187) -> (270.6639, 210.1215)
  line L4034 (270.6639, 210.1215) -> (270.7108, 209.8137)
  line L4035 (270.7108, 209.8137) -> (270.7266, 209.4968)
  line L4036 (270.7266, 209.4968) -> (270.7108, 209.1798)
  line L4037 (270.7108, 209.1798) -> (270.6639, 208.872)
  line L4038 (270.6639, 208.872) -> (270.5874, 208.575)
  line L4039 (270.5874, 208.575) -> (270.4831, 208.2901)
  line L4040 (270.4831, 208.2901) -> (270.3525, 208.0192)
  line L4041 (270.3525, 208.0192) -> (270.1975, 207.7635)
  line L4042 (270.1975, 207.7635) -> (270.019, 207.525)
  line L4043 (270.019, 207.525) -> (269.8188, 207.3048)
  line L4044 (269.8188, 207.3048) -> (269.5987, 207.1047)
  line L4045 (269.5987, 207.1047) -> (269.36, 206.9262)
  line L4046 (269.36, 206.9262) -> (269.1043, 206.771)
  line L4047 (269.1043, 206.771) -> (268.8335, 206.6404)
  line L4048 (268.8335, 206.6404) -> (268.5486, 206.5362)
  line L4049 (268.5486, 206.5362) -> (268.2517, 206.4597)
  line L4050 (268.2517, 206.4597) -> (267.9437, 206.4129)
  line L4051 (267.9437, 206.4129) -> (267.6267, 206.3969)
  line L4052 (267.6267, 206.3969) -> (267.3098, 206.4129)
  line L4053 (267.3098, 206.4129) -> (267.0021, 206.4597)
  line L4054 (267.0021, 206.4597) -> (266.7048, 206.5362)
  line L4055 (266.7048, 206.5362) -> (266.4203, 206.6404)
  line L4056 (266.4203, 206.6404) -> (266.1491, 206.771)
  line L4057 (266.1491, 206.771) -> (265.8935, 206.9262)
  line L4058 (265.8935, 206.9262) -> (265.6548, 207.1047)
  line L4059 (265.6548, 207.1047) -> (265.4346, 207.3048)
  line L4060 (265.4346, 207.3048) -> (265.2348, 207.525)
  line L4061 (265.2348, 207.525) -> (265.0563, 207.7635)
  line L4062 (265.0563, 207.7635) -> (264.901, 208.0192)
  line L4063 (264.901, 208.0192) -> (264.7704, 208.2901)
  line L4064 (264.7704, 208.2901) -> (264.666, 208.575)
  line L4065 (264.666, 208.575) -> (264.5899, 208.872)
  line L4066 (264.5899, 208.872) -> (264.5427, 209.1798)
  line L4067 (264.5427, 209.1798) -> (264.5268, 209.4968)
  line L4068 (98.6277, 148.7368) -> (111.6276, 148.7368) construction
  line L4069 (105.1278, 157.2373) -> (105.1278, 140.2364) construction
  point P0 (0, 0)
  constraints: 7828 end point, 4 midpoint, 150 other
sketch "Sketch3" plane through (0, 0, 0) normal (0, 0, 1) x (1, 0, 0)
  line L0 (-14.8739, 78.696) -> (-61.8722, 78.696) construction
  line L1 (-64.8722, 81.696) -> (-64.8722, 215.6959) construction
  line L2 (12.6874, 106.2571) -> (-14.8739, 78.696) construction
  line L3 (197.1053, 106.2571) -> (12.6874, 106.2571) construction
  line L4 (224.6664, 78.696) -> (197.1053, 106.2571) construction
  line L5 (272.1277, 78.696) -> (224.6664, 78.696) construction
  line L6 (275.1277, 215.6959) -> (275.1277, 81.696) construction
  spline S0 degree 3 poles (275.1277, 81.696) (275.1277, 80.0389) (273.7845, 78.696) (272.1277, 78.696) knots 3 3 3 3 4 4 4 4 construction
  spline S1 degree 3 poles (272.1277, 218.6959) (273.7845, 218.6959) (275.1277, 217.3526) (275.1277, 215.6959) knots 1 1 1 1 2 2 2 2 construction
  line L7 (224.6643, 218.6959) -> (272.1277, 218.6959) construction
  line L8 (197.1645, 191.1959) -> (224.6643, 218.6959) construction
  line L9 (12.6282, 191.1959) -> (197.1645, 191.1959) construction
  line L10 (-14.8718, 218.6959) -> (12.6282, 191.1959) construction
  line L11 (-61.8722, 218.6959) -> (-14.8718, 218.6959) construction
  line L12 (12.6282, 191.1959) -> (197.1645, 191.1959)
  line L13 (197.1645, 191.1959) -> (224.6643, 218.6959)
  line L14 (224.6643, 218.6959) -> (272.1277, 218.6959)
  line L15 (275.1277, 215.6959) -> (275.1277, 81.696)
  line L16 (272.1277, 78.696) -> (224.6664, 78.696)
  line L17 (224.6664, 78.696) -> (197.1053, 106.2571)
  line L18 (197.1053, 106.2571) -> (12.6874, 106.2571)
  arc A0 (272.1277, 78.696) -> (275.1277, 81.696) centre (272.1277, 81.696) ccw
  arc A1 (275.1277, 215.6959) -> (272.1277, 218.6959) centre (272.1277, 215.6959) ccw
  line L19 (105.1278, 157.2373) -> (105.1278, 140.2364) construction
  line L20 (12.6282, 191.1959) -> (-14.8718, 218.6959)
  line L21 (-14.8718, 218.6959) -> (-61.8722, 218.6959)
  line L22 (-64.8722, 215.6959) -> (-64.8722, 81.696)
  line L23 (-61.8722, 78.696) -> (-14.8739, 78.696)
  line L24 (-14.8739, 78.696) -> (12.6874, 106.2571)
  arc A2 (-64.8722, 81.696) -> (-61.8722, 78.696) centre (-61.8722, 81.696) ccw
  arc A3 (-61.8722, 218.6959) -> (-64.8722, 215.6959) centre (-61.8722, 215.6959) ccw
  point P0 (0, 0)
  constraints: 24 end point, 8 point on circle, 5 collinear, 5 tangent, 4 centre point, 2 parallel, 2 perpendicular, 2 other
extrude "Extrusion1" add sketch "Sketch3" along normal blind 2